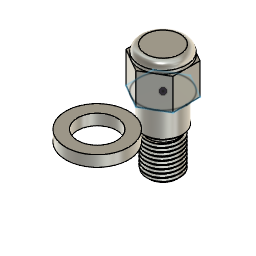
MagBolt (Autodesk Fusion 360 design; units mm, degrees)
Autodesk Fusion 360 part; units mm, degrees
sketch "Sketch1" plane through (0, 0, 0) normal (0, 0, 1) x (1, 0, 0)
  circle A0 centre (0, 0) radius 9.525
  line L0 (9.525, 5.4993) -> (0, 10.9985)
  line L1 (0, 10.9985) -> (-9.525, 5.4993)
  line L2 (-9.525, 5.4993) -> (-9.525, -5.4993)
  line L3 (-9.525, -5.4993) -> (0, -10.9985)
  line L4 (0, -10.9985) -> (9.525, -5.4993)
  line L5 (9.525, -5.4993) -> (9.525, 5.4993)
  dimension "d1" = 19.05
  constraint coincident A0.centre origin
  measures "d1" diameter of A0
extrude "Extrude1" add sketch "Sketch1" along normal blind 12.7 makes body 1
extrude "Extrude2" add sketch "Sketch1" along normal blind 16.51 contours A0 bodies 1
sketch "Sketch2" plane through (0, 0, 0) normal (0, 0, 1) x (1, 0, 0)
  circle A0 centre (0, 0) radius 7.9375
  dimension "d6" = 15.875
  constraint coincident A0.centre origin
  measures "d6" diameter of A0
extrude "Extrude3" add sketch "Sketch2" against normal blind 12.065 bodies 1
chamfer "Chamfer1" distance 0.7937 angle 45 1 edges at (-7.4003, 2.8703, -12.065) on bodies 1
sketch "Sketch3" plane through (0, 0, -12.065) normal (0, 0, -1) x (1, 0, 0)
  circle A0 centre (0, 0) radius 7.1437
  circle A1 centre (0, 0) radius 6.0545
  dimension "d10" = 12.1089
  constraint coincident A0.centre A1.centre
  measures "d10" diameter of A1
extrude "Extrude4" add sketch "Sketch3" along normal blind 1.5875 contours A1 bodies 1
sketch "Sketch4" plane through (0, 0, -13.6525) normal (0, 0, -1) x (1, 0, 0)
  circle A0 centre (0, 0) radius 6.0545
  circle A1 centre (0, 0) radius 6.7469
  dimension "d15" = 13.4938
  constraint coincident A0.centre A1.centre
  measures "d15" diameter of A1
extrude "Extrude5" add sketch "Sketch4" along normal blind 14.2875 contours A0 | A1 bodies 1
thread "Thread2" "ISO Metric profile 14.0 M14x1.5 6g" major diameter 13.85 minor diameter 12.137 pitch 1.5 angle 60 modelled right hand crest width 0.2154 on face at (6.7385, 0.3363, -23.1775) from (0, 0, -13.6525) to (0, 0, -27.686) crest through (6.925, 0, -13.2775) on bodies 1
chamfer "Chamfer2" distance 1.143 angle 45 1 edges at (-6.4564, 2.5042, -27.94) on bodies 1
fillet "Fillet1" radius 2.54 1 edges at (-8.8804, -3.4444, 16.51) on bodies 1
sketch "Sketch6" plane through (0, 0, 0) normal (0, 0, 1) x (1, 0, 0)
  circle A0 centre (0, 0) radius 7.9375
  circle A1 centre (0, 0) radius 12.7
  dimension "d26" = 15.875
  dimension "d27" = 25.4
  constraint coincident A0.centre A1.centre
  measures "d26" diameter of A0
  measures "d27" diameter of A1
extrude "Extrude6" add sketch "Sketch6" along normal blind 4.445 separate body makes body 2
move_body "Move1" bodies 2 to x (1, 0, 0) y (0, 1, 0) z (0, 0, 1) at (0, 0, -4.445)
move_body "Move2" bodies 2 to x (1, 0, 0) y (0, 1, 0) z (0, 0, 1) at (0, -26.67, 0)
equation "d9 = ( 1 / 32 ) * 1 in"
equation "d11 = ( 1 / 16 ) * 1 in"
equation "d15 = ( 17 / 32 ) * 1 in"
equation "d16 = ( ( 5 / 8 ) * 1 in ) - ( ( 4 / 64 ) * 1 in )"
named bodies: "Bolt", "Washer"
